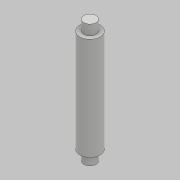
# Autodesk Inventor part: exercise2-6
Saved by Autodesk Inventor 2018 (Build 220112000, 112)
## iProperties
Created: 2020-09-21
Part Number: exercise2-6
Material: 一般
Document SubType Name: Modeling
Designer: 王鼎鈞
Density: 1 g/cm^3
Appearance: 預設
Author: 王鼎鈞
Autodesk Inventor part; units mm, degrees
ref_plane "YZ Plane" through (0, 0, 0) normal (1, 0, 0) x (0, 1, 0)
ref_plane "XZ Plane" through (0, 0, 0) normal (0, 1, 0) x (-1, 0, 0)
ref_plane "XY Plane" through (0, 0, 0) normal (0, 0, 1) x (1, 0, 0)
sketch "草圖1" plane through (0, 0, 0) normal (1, 0, 0) x (0, 1, 0)
  line L0 (-2, 0) -> (12, 0) projected
  line L1 (0, -134) -> (0, 34) projected
  line L2 (0, 0) -> (10, 0)
  line L3 (10, 0) -> (10, -100)
  line L4 (10, -100) -> (0, -100)
  line L5 (0, -100) -> (0, 0)
  line L6 (0, -100) -> (6, -100)
  line L7 (6, -100) -> (6, -110)
  line L8 (6, -110) -> (0, -110)
  line L9 (0, -110) -> (0, -100)
  line L10 (0, 0) -> (6, 0)
  line L11 (6, 0) -> (6, 10)
  line L12 (6, 10) -> (0, 10)
  line L13 (0, 10) -> (0, 0)
  dimension "d0" = 10
  dimension "d1" = 100
  dimension "d2" = 6
  dimension "d3" = 10
  dimension "d4" = 6
  dimension "d5" = 10
  constraints: 24 end point, 6 parallel, 3 horizontal, 3 perpendicular
  measures "d0" distance of L3.end L4.end
  measures "d1" distance of L2.end L3.end
  measures "d2" distance of L7.end L8.end
  measures "d3" distance of L6.end L7.end
  measures "d4" distance of L12.end L11.end
  measures "d5" distance of L11.end L10.end
revolve "迴轉1" add sketch "草圖1" angle 360 about axis through (0, 0, -100) along (0, 0, 1)
